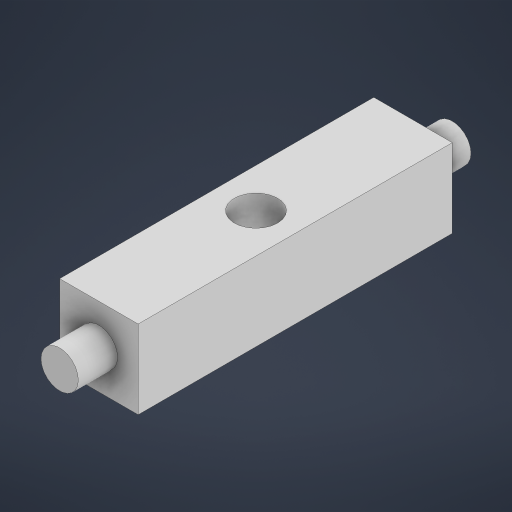
# Autodesk Inventor part: FP V2 Arm Connector
Saved by Autodesk Inventor 2023.6 (Build 276521000, 521)
## iProperties
Created: 2026-02-19
Part Number: FP V2 Arm Connector
Material: Generic
Document SubType Name: Modeling
Designer: user
Density: 1 g/cm^3
Appearance: Default
Author: user
Autodesk Inventor part; units mm, degrees
ref_plane "YZ Plane" through (0, 0, 0) normal (1, 0, 0) x (0, 1, 0)
sketch "Sketch1" plane through (0, 0, 0) normal (0, 0, 1) x (1, 0, 0)
  line L0 (-10, 10) -> (10, 10)
  line L1 (10, 10) -> (10, -10)
  line L2 (10, -10) -> (-10, -10)
  line L3 (-10, -10) -> (-10, 10)
  line L4 (-10, 10) -> (10, -10) construction
  line L5 (10, 10) -> (-10, -10) construction
  point P0 (0, 0)
  dimension "d0" = 20
  dimension "d1" = 20
  constraints: 12 end point, 2 midpoint, 2 parallel, 1 horizontal, 1 perpendicular
  measures "d0" distance between parallel lines of L1 L3
  measures "d1" distance between parallel lines of L0 L2
extrude "Extrusion1" add sketch "Sketch1" along normal blind 80
sketch "Sketch2" plane through (0, 0, 80) normal (0, 0, 1) x (1, 0, 0)
  circle A0 centre (0, 0) radius 4.75
  dimension "d4" = 9.5
  constraints: 1 centre point, 1 coincident
  measures "d4" diameter of A0
extrude "Extrusion2" add sketch "Sketch2" along normal blind 10
ref_plane "Work Plane1" through (0, 0, 40) normal (0, 0, 1) x (1, 0, 0)
mirror "Mirror1" about plane through (0, 0, 40) normal (0, 0, 1) of "Extrusion2"
ref_plane "Work Plane2" through (-8, 10, 0) normal (0, 1, 0) x (1, 0, 0)
sketch "Sketch3" plane through (-8, 10, 0) normal (0, 1, 0) x (1, 0, 0)
  line L0 (-2, -80) -> (-2, 0) projected
  line L1 (-2, -40) -> (18, -40)
  line L2 (18, 0) -> (18, -80) projected
  circle A0 centre (8, -40) radius 5.5
  point P0 (8, 0)
  dimension "d8" = 11
  constraints: 3 midpoint, 2 end point, 1 centre point
  measures "d8" diameter of A0
extrude "Extrusion3" cut sketch "Sketch3" against normal through all
body "Solid1"
